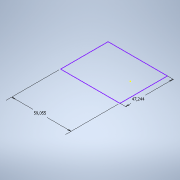
# Autodesk Inventor part: placa22
Saved by Autodesk Inventor 2021 (Build 250183000, 183)
## iProperties
Created: 2021-03-18
Part Number: placa22
Material: Steel, Carbon
Document SubType Name: Modeling
Designer: andre
Density: 7.85 g/cm^3
Appearance: Semi-Polished
Author: andre
Autodesk Inventor part; units mm, degrees
ref_plane "YZ Plane" through (0, 0, 0) normal (1, 0, 0) x (0, 1, 0)
ref_plane "XZ Plane" through (0, 0, 0) normal (0, 1, 0) x (-1, 0, 0)
ref_plane "XY Plane" through (0, 0, 0) normal (0, 0, 1) x (1, 0, 0)
sketch "Sketch1" plane through (0, 0, 0) normal (0, 1, 0) x (-1, 0, 0)
  line L0 (1305.3571, 614.2857) -> (-344.6429, 614.2857)
  line L1 (-344.6429, 614.2857) -> (-344.6429, -553.7143)
  line L2 (-344.6429, -553.7143) -> (1305.3571, -553.7143)
  line L3 (1305.3571, -553.7143) -> (1305.3571, 614.2857)
  point P0 (0, 0)
  dimension "d0" = 1168
  dimension "d1" = 1650
  constraints: 8 end point, 2 parallel, 1 horizontal, 1 perpendicular
  measures "d0" distance of L0.end L1.end
  measures "d1" distance of L0.start L0.end
extrude "Extrusion1" add sketch "Sketch1" along normal blind 12.7
body "Solid1"
